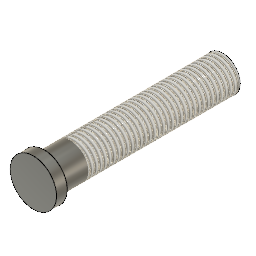
_spindle.bfd7bfdf-98ad-41ff-92fa-3afda45fb48c (Autodesk Fusion 360 design; units mm, degrees)
Autodesk Fusion 360 part; units mm, degrees
sketch "Sketch1" plane through (0, 0, 0) normal (0, 1, 0) x (1, 0, 0)
  circle A0 centre (0, 0) radius 13
  dimension "d1" = 26
  constraint coincident A0.centre origin
  measures "d1" diameter of A0
extrude "Extrude1" add sketch "Sketch1" along normal blind 6
sketch "Sketch2" plane through (0, 6, 0) normal (0, 1, 0) x (-1, 0, 0)
  circle A0 centre (0, 0) radius 13
  circle A1 centre (0, 0) radius 10
  dimension "d4" = 20
  constraint coincident A0.centre A1.centre
  measures "d4" diameter of A1
extrude "Extrude2" add sketch "Sketch2" along normal blind 100 contours A1
thread "Thread1" "ISO Metric profile 20.0 M20x2.5 6g" major diameter 19.7905 minor diameter 16.938 pitch 2.5 angle 60 resizes the face on face at (-9.9503, 39.3333, -0.9957) from (0, 21, 0) to (0, 106, 0)
